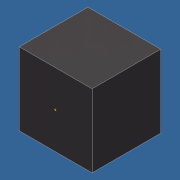
# Autodesk Inventor part: Modul Gehäuse
Saved by Autodesk Inventor 2018.2 (Build 222227000, 227)
## iProperties
Created: 2018-10-15
Part Number: Modul Gehäuse
Material: CFK
Document SubType Name: Modeling
Designer: N.Grubert
Density: 1.43 g/cm^3
Appearance: Kohlenstofffaser
Fläche: 0 cm²
Gewicht: 0 g
Material: geeigneten Werkstoff auswählen !
Dateiname: P:\INVENTOR\Inventor 2018\Templates\ILT\Norm.ipt
Bez_eng: bolt
Bez_french: boulon
Author: N.Grubert
Autodesk Inventor part; units mm, degrees
ref_plane "YZ Plane" through (0, 0, 0) normal (1, 0, 0) x (0, 1, 0)
ref_plane "XZ Plane" through (0, 0, 0) normal (0, 1, 0) x (-1, 0, 0)
ref_plane "XY Plane" through (0, 0, 0) normal (0, 0, 1) x (1, 0, 0)
sketch "Skizze4" plane through (0, 0, 0) normal (0, 1, 0) x (-1, 0, 0)
  line L0 (26.5, 26.5) -> (-26.5, 26.5)
  line L1 (-26.5, 26.5) -> (-26.5, -26.5)
  line L2 (-26.5, -26.5) -> (26.5, -26.5)
  line L3 (26.5, -26.5) -> (26.5, 26.5)
  line L4 (37.1, 0) -> (-37.1, 0) construction
  line L5 (0, -37.1) -> (0, 37.1) construction
  point P0 (0, 0)
  dimension "d4" = 53
  dimension "d5" = 53
  constraints: 8 end point, 2 parallel, 1 horizontal, 1 perpendicular, 2 other
  measures "d4" distance of L0.end L1.end
  measures "d5" distance between parallel lines of L3 L1
extrude "Extrusion2" add sketch "Skizze4" along normal blind 5
sketch "Skizze5" plane through (0, 5, 0) normal (0, 1, 0) x (1, 0, 0)
  line L0 (-26.5, -26.5) -> (26.5, -26.5) projected
  line L1 (26.5, -26.5) -> (26.5, 26.5) projected
  line L2 (26.5, 26.5) -> (-26.5, 26.5) projected
  line L3 (-26.5, 26.5) -> (-26.5, -26.5) projected
  line L4 (-24, -24) -> (24, -24)
  line L5 (24, -24) -> (24, 24)
  line L6 (24, 24) -> (-24, 24)
  line L7 (-24, 24) -> (-24, -24)
  point P0 (0, 0)
  dimension "d8" = 2.5
  constraints: 8 end point, 3 other
  measures "d8" distance between parallel lines of L7 L3
extrude "Extrusion3" add sketch "Skizze5" along normal blind 45
